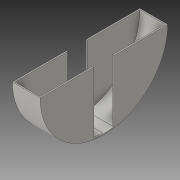
# Autodesk Inventor part: GearHolster
Saved by Autodesk Inventor 2016 (Build 200138000, 138)
## iProperties
Created: 2017-01-10
Part Number: GearHolster
Material: Generic
Document SubType Name: Modeling
Designer: hamblettk
Density: 1 g/cm^3
Appearance: Default
Author: hamblettk
Autodesk Inventor part; units mm, degrees
ref_plane "YZ Plane" through (0, 0, 0) normal (1, 0, 0) x (0, 1, 0)
ref_plane "XZ Plane" through (0, 0, 0) normal (0, 1, 0) x (-1, 0, 0)
ref_plane "XY Plane" through (0, 0, 0) normal (0, 0, 1) x (1, 0, 0)
sketch "Sketch1" plane through (0, 0, 0) normal (1, 0, 0) x (0, 1, 0)
  line L0 (0, 0) -> (0, -292.1)
  arc A0 (0, 0) -> (0, -292.1) centre (0, -146.05) ccw
  dimension "d0" = 292.1
  dimension "d1" = 146.05
  constraints: 2 end point, 2 point on circle, 1 centre point, 1 vertical
  measures "d0" distance of L0.start L0.end
  measures "d1" radius of A0
extrude "Extrusion1" add sketch "Sketch1" along normal blind 63.5
shell "Shell1" thickness 2.54 removed faces 1 at (42.3333, 0, -97.3667)
sketch "Sketch3" plane through (63.5, 0, 0) normal (1, 0, 0) x (0, 0, -1)
  line L0 (292.1, 0) -> (0, 0) projected
  line L1 (123.4186, 0) -> (168.6814, 0)
  line L2 (123.4186, 0) -> (123.4186, -144.4974)
  line L3 (168.6814, 0) -> (168.6814, -144.4974)
  arc A0 (2.54, 0) -> (289.56, 0) centre (146.05, 0) ccw projected
  arc A1 (123.4186, -141.5071) -> (168.6814, -141.7143) centre (146.663, -7.7251) ccw
  dimension "d9" = 45.2628
  dimension "d10" = 123.4186
  constraints: 6 end point, 4 point on line, 3 point on circle, 2 vertical, 1 centre point
  measures "d9" distance of L1.start L1.end
  measures "d10" distance of L0.end L1.start
extrude "Extrusion4" cut sketch "Sketch3" against normal blind 3810000 contours L3 A0 A1 L2 L0 | A1 A0
body "Solid1"
